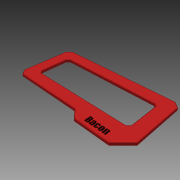
# Autodesk Inventor part: display_2004_frame
Saved by Autodesk Inventor 2014 (Build 180170000, 170)
## iProperties
Created: 2014-01-22
Part Number: display_2004_frame
Material: ABS Plastic
Document SubType Name: Modeling
Designer: buben
Density: 1.06 g/cm^3
Appearance: Light Red
Author: buben
Autodesk Inventor part; units mm, degrees
ref_plane "YZ Plane" through (0, 0, 0) normal (1, 0, 0) x (0, 1, 0)
ref_plane "XZ Plane" through (0, 0, 0) normal (0, 1, 0) x (-1, 0, 0)
ref_plane "XY Plane" through (0, 0, 0) normal (0, 0, 1) x (1, 0, 0)
sketch "Sketch1" plane through (0, 0, 0) normal (0, 1, 0) x (-1, 0, 0)
  line L0 (2, 0) -> (78, 0)
  line L1 (80, 2) -> (80, 25)
  line L2 (78, 27) -> (2, 27)
  line L3 (0, 25) -> (0, 2)
  line L4 (0, 25) -> (2, 27)
  line L5 (78, 27) -> (80, 25)
  line L6 (80, 2) -> (78, 0)
  line L7 (2, 0) -> (0, 2)
  line L8 (-6, 37) -> (86, 37)
  line L9 (90, 33) -> (90, -6)
  line L10 (86, -10) -> (-6, -10)
  line L11 (-10, -6) -> (-10, 33)
  line L12 (-10, 33) -> (-6, 37)
  line L13 (86, 37) -> (90, 33)
  line L14 (90, -6) -> (86, -10)
  line L15 (-6, -10) -> (-10, -6)
  point P0 (0, 0)
  point P1 (80, 27)
  point P2 (80, 0)
  point P3 (0, 27)
  point P4 (-10, 37)
  point P5 (90, -10)
  point P6 (90, 37)
  point P7 (-10, -10)
  point P8 (40, 37)
  point P9 (40, 27)
  point P10 (-10, 13.5)
  point P11 (0, 13.5)
  dimension "d0" = 2
  dimension "d1" = 2
  dimension "d2" = 2
  dimension "d3" = 2
  dimension "d4" = 2
  dimension "d5" = 2
  dimension "d6" = 2
  dimension "d7" = 2
  dimension "d8" = 80
  dimension "d9" = 27
  dimension "d10" = 4
  dimension "d11" = 4
  dimension "d12" = 4
  dimension "d13" = 4
  dimension "d14" = 4
  dimension "d15" = 4
  dimension "d16" = 4
  dimension "d17" = 4
  dimension "d18" = 10
  dimension "d19" = 10
  constraints: 32 end point, 16 point on line, 4 midpoint, 4 parallel, 2 horizontal, 2 perpendicular, 1 horizontal alignment, 1 vertical alignment
  measures "d0" distance of L3.start point (0, 27)
  measures "d1" distance of L2.end point (0, 27)
  measures "d2" distance of L2.start point (80, 27)
  measures "d3" distance of L1.end point (80, 27)
  measures "d4" distance of L1.start point (80, 0)
  measures "d5" distance of L0.end point (80, 0)
  measures "d6" distance of L0.start point (0, 0)
  measures "d7" distance of L3.end point (0, 0)
  measures "d8" distance between parallel lines of L1 L3
  measures "d9" distance between parallel lines of L0 L2
  measures "d10" distance of L11.end point (-10, 37)
  measures "d11" distance of L8.start point (-10, 37)
  measures "d12" distance of L8.end point (90, 37)
  measures "d13" distance of L9.start point (90, 37)
  measures "d14" distance of L9.end point (90, -10)
  measures "d15" distance of L10.start point (90, -10)
  measures "d16" distance of L10.end point (-10, -10)
  measures "d17" distance of L11.start point (-10, -10)
  measures "d18" distance between parallel lines of L3 L11
  measures "d19" distance between parallel lines of L2 L8
extrude "Extrusion1" add sketch "Sketch1" along normal blind 2
sketch "Sketch2" plane through (0, 2, 0) normal (0, 1, 0) x (1, 0, 0)
  line L0 (-90, -33) -> (-86, -37) projected
  line L1 (-86, -37) -> (6, -37) projected
  line L2 (6, -37) -> (0, -43)
  line L3 (0, -43) -> (-26, -43)
  line L4 (-26, -43) -> (-32, -37)
  point P0 (0, 0)
  dimension "d22" = 6
  dimension "d23" = 26
  constraints: 6 end point, 2 perpendicular, 1 parallel, 1 point on line
  measures "d22" distance between parallel lines of L1 L3
  measures "d23" distance of L2.end L3.end
extrude "Extrusion2" add sketch "Sketch2" against normal blind 2
chamfer "Chamfer1" distance 0.3 angle 45 18 edges at (-80, 2, 13.5) (-79, 2, 26) (-40, 2, 27) (-79, 2, 1) (-40, 2, 0) (-1, 2, 26) (0, 2, 13.5) (-1, 2, 1) (5, 2, 38) (10, 2, 13.5) (8, 2, -8) (-13, 2, 43) (-29, 2, 40) (-59, 2, 37) (-88, 2, 35) (-90, 2, 13.5) (-88, 2, -8) (-40, 2, -10)
sketch "Sketch3" plane through (0, 2, 0) normal (0, 1, 0) x (1, 0, 0)
  line L0 (-25.8757, -42.7) -> (-31.8757, -36.7) projected
  line L1 (-0.1243, -42.7) -> (-25.8757, -42.7) projected
  line L2 (9.7, -32.8757) -> (-0.1243, -42.7) projected
  line L3 (-31.8757, -36.7) -> (-85.8757, -36.7) projected
  line L4 (-23, -35.2) -> (-3, -35.2) construction
  line L5 (-3, -35.2) -> (-3, -40.2) construction
  line L6 (-3, -40.2) -> (-23, -40.2) construction
  line L7 (-23, -40.2) -> (-23, -35.2) construction
  line L8 (-23, -37.7) -> (-30.8757, -37.7) construction
  line L9 (-3, -37.7) -> (4.8757, -37.7) construction
  line L10 (-20.9145, -35.2) -> (-19.6183, -35.2)
  spline S0 degree 2 poles (-19.6183, -35.2) (-19.0004, -35.2) (-18.3674, -35.3922) (-17.9793, -35.9762) (-17.9793, -36.6243) knots 0 0 0 1 2 3 3 3
  spline S1 degree 2 poles (-17.9793, -36.6243) (-17.9793, -37.0613) (-18.2543, -37.408) (-18.6613, -37.4984) knots 0 0 0 1 2 2 2
  spline S2 degree 2 poles (-18.6613, -37.4984) (-18.2091, -37.6039) (-17.8888, -38.0749) (-17.8888, -38.5647) knots 0 0 0 1 2 2 2
  line L11 (-17.8888, -38.5647) -> (-17.8888, -39.0244)
  spline S3 degree 2 poles (-17.8888, -39.0244) (-17.8888, -39.5331) (-18.1187, -40.0191) (-18.6274, -40.2) (-19.4111, -40.2) knots 0 0 0 1 2 3 3 3
  line L12 (-19.4111, -40.2) -> (-20.9145, -40.2)
  line L13 (-20.9145, -40.2) -> (-20.9145, -35.2)
  line L14 (-19.6145, -37.9468) -> (-19.6145, -39.3447)
  spline S4 degree 2 poles (-19.6145, -39.3447) (-19.3395, -39.3372) (-19.1888, -39.1827) (-19.1888, -38.8775) knots 0 0 0 1 2 2 2
  line L15 (-19.1888, -38.8775) -> (-19.1888, -38.414)
  spline S5 degree 2 poles (-19.1888, -38.414) (-19.1888, -38.09) (-19.3244, -37.9543) (-19.6145, -37.9468) knots 0 0 0 1 2 2 2
  line L16 (-19.6145, -36.0553) -> (-19.6145, -37.1668)
  spline S6 degree 2 poles (-19.6145, -37.1668) (-19.5317, -37.1631) (-19.4864, -37.1631) knots 0 0 0 1 1 1
  spline S7 degree 2 poles (-19.4864, -37.1631) (-19.2943, -37.1631) (-19.1888, -36.9747) (-19.1888, -36.5301) knots 0 0 0 1 2 2 2
  spline S8 degree 2 poles (-19.1888, -36.5301) (-19.1888, -36.2965) (-19.2754, -36.1081) (-19.4148, -36.0591) (-19.6145, -36.0553) knots 0 0 0 1 2 3 3 3
  line L17 (-16.344, -37.6868) -> (-17.5158, -37.6868)
  line L18 (-17.5158, -37.6868) -> (-17.5158, -37.4118)
  spline S9 degree 2 poles (-17.5158, -37.4118) (-17.5158, -36.937) (-17.2973, -36.4208) (-16.6341, -36.0252) (-16.1066, -36.0252) knots 0 0 0 1 2 3 3 3
  spline S10 degree 2 poles (-16.1066, -36.0252) (-15.4736, -36.0252) (-14.8293, -36.4735) (-14.7012, -37.1254) (-14.7012, -38.1427) knots 0 0 0 1 2 3 3 3
  line L19 (-14.7012, -38.1427) -> (-14.7012, -40.2)
  line L20 (-14.7012, -40.2) -> (-15.9145, -40.2)
  line L21 (-15.9145, -40.2) -> (-15.9145, -39.8345)
  spline S11 degree 2 poles (-15.9145, -39.8345) (-16.0275, -40.0531) (-16.3892, -40.2754) (-16.6417, -40.2754) knots 0 0 0 1 2 2 2
  spline S12 degree 2 poles (-16.6417, -40.2754) (-16.9695, -40.2754) (-17.5158, -39.9061) (-17.5158, -39.2844) knots 0 0 0 1 2 2 2
  line L22 (-17.5158, -39.2844) -> (-17.5158, -38.9491)
  spline S13 degree 2 poles (-17.5158, -38.9491) (-17.5158, -38.4894) (-17.2257, -38.154) (-16.6492, -37.9317) knots 0 0 0 1 2 2 2
  spline S14 degree 2 poles (-16.6492, -37.9317) (-16.035, -37.6906) (-15.9484, -37.5248) (-15.9484, -37.2686) knots 0 0 0 1 2 2 2
  spline S15 degree 2 poles (-15.9484, -37.2686) (-15.9484, -36.9483) (-16.0426, -36.7524) (-16.1556, -36.7524) knots 0 0 0 1 2 2 2
  spline S16 degree 2 poles (-16.1556, -36.7524) (-16.2837, -36.7524) (-16.344, -36.9144) (-16.344, -37.2573) knots 0 0 0 1 2 2 2
  line L23 (-16.344, -37.2573) -> (-16.344, -37.6868)
  spline S17 degree 2 poles (-15.9484, -38.2482) (-16.2498, -38.4668) (-16.344, -38.7644) (-16.344, -39.0433) knots 0 0 0 1 2 2 2
  spline S18 degree 2 poles (-16.344, -39.0433) (-16.344, -39.3635) (-16.2611, -39.5482) (-16.1368, -39.5482) knots 0 0 0 1 2 2 2
  spline S19 degree 2 poles (-16.1368, -39.5482) (-16.02, -39.5482) (-15.9484, -39.4012) (-15.9484, -39.0922) knots 0 0 0 1 2 2 2
  line L24 (-15.9484, -39.0922) -> (-15.9484, -38.2482)
  line L25 (-11.5136, -37.6491) -> (-12.6891, -37.6491)
  line L26 (-12.6891, -37.6491) -> (-12.6891, -37.1744)
  spline S20 degree 2 poles (-12.6891, -37.1744) (-12.6891, -36.9295) (-12.7683, -36.7524) (-12.8775, -36.7524) knots 0 0 0 1 2 2 2
  spline S21 degree 2 poles (-12.8775, -36.7524) (-12.9868, -36.7524) (-13.0622, -36.9069) (-13.0622, -37.1744) knots 0 0 0 1 2 2 2
  line L27 (-13.0622, -37.1744) -> (-13.0622, -39.1111)
  spline S22 degree 2 poles (-13.0622, -39.1111) (-13.0622, -39.3296) (-12.9491, -39.5482) (-12.8436, -39.5482) knots 0 0 0 1 2 2 2
  spline S23 degree 2 poles (-12.8436, -39.5482) (-12.7155, -39.5482) (-12.6251, -39.3183) (-12.6251, -39.0018) knots 0 0 0 1 2 2 2
  line L28 (-12.6251, -39.0018) -> (-12.6251, -38.5157)
  line L29 (-12.6251, -38.5157) -> (-11.5136, -38.5157)
  spline S24 degree 2 poles (-11.5136, -38.5157) (-11.5173, -39.0056) (-11.5814, -39.4992) (-11.9318, -40.0116) (-12.4932, -40.2754) (-12.9077, -40.2754) knots 0 0 0 1 2 3 4 4 4
  spline S25 degree 2 poles (-12.9077, -40.2754) (-13.4352, -40.2754) (-14.0531, -39.9136) (-14.3093, -39.2618) (-14.3093, -38.6627) knots 0 0 0 1 2 3 3 3
  line L30 (-14.3093, -38.6627) -> (-14.3093, -37.4946)
  spline S26 degree 2 poles (-14.3093, -37.4946) (-14.3093, -36.9747) (-14.0983, -36.4434) (-13.4126, -36.0252) (-12.9228, -36.0252) knots 0 0 0 1 2 3 3 3
  spline S27 degree 2 poles (-12.9228, -36.0252) (-12.4329, -36.0252) (-11.7434, -36.4396) (-11.5136, -37.0689) (-11.5136, -37.6491) knots 0 0 0 1 2 3 3 3
  line L31 (-8.3222, -37.5399) -> (-8.3222, -38.5459)
  spline S28 degree 2 poles (-8.3222, -38.5459) (-8.3222, -39.096) (-8.4314, -39.6122) (-8.7969, -40.0606) (-9.3696, -40.2754) (-9.7389, -40.2754) knots 0 0 0 1 2 3 4 4 4
  spline S29 degree 2 poles (-9.7389, -40.2754) (-10.1534, -40.2754) (-10.7298, -40.0945) (-11.0463, -39.7252) (-11.182, -39.2015) (-11.182, -38.6815) knots 0 0 0 1 2 3 4 4 4
  line L32 (-11.182, -38.6815) -> (-11.182, -37.6303)
  spline S30 degree 2 poles (-11.182, -37.6303) (-11.182, -37.0576) (-10.9333, -36.4133) (-10.2928, -36.0252) (-9.7916, -36.0252) knots 0 0 0 1 2 3 3 3
  spline S31 degree 2 poles (-9.7916, -36.0252) (-9.3734, -36.0252) (-8.7705, -36.2739) (-8.4427, -36.677) (-8.3222, -37.1028) (-8.3222, -37.5399) knots 0 0 0 1 2 3 4 4 4
  spline S32 degree 2 poles (-9.5693, -37.2309) (-9.5693, -36.9144) (-9.6372, -36.7524) (-9.7502, -36.7524) knots 0 0 0 1 2 2 2
  spline S33 degree 2 poles (-9.7502, -36.7524) (-9.8595, -36.7524) (-9.9348, -36.9144) (-9.9348, -37.2309) knots 0 0 0 1 2 2 2
  line L33 (-9.9348, -37.2309) -> (-9.9348, -39.0809)
  spline S34 degree 2 poles (-9.9348, -39.0809) (-9.9348, -39.3711) (-9.8595, -39.5482) (-9.7502, -39.5482) knots 0 0 0 1 2 2 2
  spline S35 degree 2 poles (-9.7502, -39.5482) (-9.6409, -39.5482) (-9.5693, -39.3861) (-9.5693, -39.1224) knots 0 0 0 1 2 2 2
  line L34 (-9.5693, -39.1224) -> (-9.5693, -37.2309)
  line L35 (-6.6417, -36.1005) -> (-6.6643, -36.4773)
  spline S36 degree 2 poles (-6.6643, -36.4773) (-6.5286, -36.2512) (-6.1368, -36.0252) (-5.8806, -36.0252) knots 0 0 0 1 2 2 2
  spline S37 degree 2 poles (-5.8806, -36.0252) (-5.5565, -36.0252) (-5.1496, -36.3266) (-5.0328, -36.7901) (-5.0328, -37.3251) knots 0 0 0 1 2 3 3 3
  line L36 (-5.0328, -37.3251) -> (-5.0328, -40.2)
  line L37 (-5.0328, -40.2) -> (-6.28, -40.2)
  line L38 (-6.28, -40.2) -> (-6.28, -37.3628)
  spline S38 degree 2 poles (-6.28, -37.3628) (-6.28, -36.937) (-6.3365, -36.7524) (-6.4646, -36.7524) knots 0 0 0 1 2 2 2
  spline S39 degree 2 poles (-6.4646, -36.7524) (-6.5965, -36.7524) (-6.6643, -36.9671) (-6.6643, -37.4306) knots 0 0 0 1 2 2 2
  line L39 (-6.6643, -37.4306) -> (-6.6643, -40.2)
  line L40 (-6.6643, -40.2) -> (-7.9115, -40.2)
  line L41 (-7.9115, -40.2) -> (-7.9115, -36.1005)
  line L42 (-7.9115, -36.1005) -> (-6.6417, -36.1005)
  point P0 (0, 0)
  dimension "d29" = 20
  dimension "d30" = 5
  dimension "d31" = 6
  dimension "d32" = 5
  constraints: 4 end point, 3 collinear, 2 midpoint, 2 parallel, 2 point on line, 2 other
  measures "d29" distance of L4.start L4.end
  measures "d30" distance of L6.end L4.start
  measures "d31" distance between parallel lines of L3 L1
  measures "d32" distance between parallel lines of L1 L8
extrude "Extrusion3" cut sketch "Sketch3" against normal blind 0.3
equation "\"d1\" = d0"
equation "\"d2\" = d0"
equation "\"d3\" = d2"
equation "\"d4\" = d0"
equation "\"d5\" = d4"
equation "\"d6\" = d0"
equation "\"d7\" = d6"
equation "\"d11\" = d10"
equation "\"d12\" = d10"
equation "\"d13\" = d12"
equation "\"d14\" = d10"
equation "\"d15\" = d14"
equation "\"d16\" = d10"
equation "\"d17\" = d16"
equation "\"d19\" = d18"
body "Solid1"
